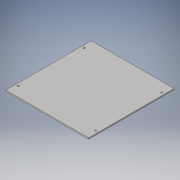
# Autodesk Inventor part: BottomPlate
Saved by Autodesk Inventor 2016 (Build 200138000, 138)
## iProperties
Created: 2015-08-06
Part Number: BottomPlate
Material: Generic
Document SubType Name: Modeling
Designer: lachesis
Density: 1 g/cm^3
Appearance: Default
Author: lachesis
Autodesk Inventor part; units mm, degrees
ref_plane "YZ Plane" through (0, 0, 0) normal (1, 0, 0) x (0, 1, 0)
ref_plane "XZ Plane" through (0, 0, 0) normal (0, 1, 0) x (-1, 0, 0)
ref_plane "XY Plane" through (0, 0, 0) normal (0, 0, 1) x (1, 0, 0)
sketch "Sketch1" plane through (0, 0, 0) normal (0, 1, 0) x (-1, 0, 0)
  line L0 (98.0186, -101.2063) -> (-98.0186, -101.2063)
  line L1 (-98.0186, -101.2063) -> (-98.0186, 101.2063)
  line L2 (-98.0186, 101.2063) -> (98.0186, 101.2063)
  line L3 (98.0186, 101.2063) -> (98.0186, -101.2063)
  point P0 (0, 0)
  point P1 (0, -101.2063)
  point P2 (98.0186, 0)
  dimension "d0" = 196.0372
  dimension "d1" = 202.4126
  constraints: 8 end point, 2 midpoint, 2 parallel, 1 horizontal, 1 horizontal alignment, 1 perpendicular, 1 vertical alignment
  measures "d0" distance of L0.start L0.end
  measures "d1" distance of L2.end L0.start
extrude "Extrusion1" add sketch "Sketch1" along normal blind 3
sketch "Sketch2" plane through (0, 3, 0) normal (0, 1, 0) x (1, 0, 0)
  line L0 (-91.6686, 78.0923) -> (91.6686, 78.0923)
  line L1 (91.6686, 78.0923) -> (91.6686, -78.0923)
  point P0 (0, 0)
  point P1 (-91.6686, -78.0923)
  point P2 (0, 78.0923)
  point P3 (91.6686, 0)
  dimension "d4" = 183.3372
  dimension "d5" = 156.1846
  constraints: 4 end point, 3 horizontal alignment, 3 vertical alignment, 2 midpoint, 1 horizontal, 1 perpendicular
  measures "d4" distance of L0.end L0.start
  measures "d5" distance of point (-91.669, -78.092) L0.start
hole "Hole1" at (-91.6686, 3, -78.0923) at (91.6686, 3, -78.0923) at (91.6686, 3, 78.0923) at (-91.6686, 3, 78.0923) direction (0, -1, 0) diameter 3.81 end through all
body "Solid1"
